Wheel Motor Support   FrontBack (Autodesk Fusion 360 design; units mm, degrees)
Autodesk Fusion 360 part; units mm, degrees
note: some values were not read from the file. Chosen so that the rebuilt part matches the saved one: which pieces of a blend or face edit are solid. Set by a fixed rule: which sketch regions a step uses.
sketch "Sketch1" plane through (0, 0, 0) normal (0, 0, 1) x (1, 0, 0)
  circle A0 centre (0, 0) radius 15.5 construction
  circle A1 centre (0, 0) radius 18.9
  circle A2 centre (0, 0) radius 20.9
  line L0 (-18.9, 0) -> (18.9, 0) construction
  circle A3 centre (-15.5, 0) radius 1.6
  circle A4 centre (15.5, 0) radius 1.6
  circle A5 centre (7.75, -13.4234) radius 1.6
  circle A6 centre (-7.75, -13.4234) radius 1.6
  circle A7 centre (7.75, 13.4234) radius 1.6
  circle A8 centre (-7.75, 13.4234) radius 1.6
  line L1 (0, 18.9) -> (0, -19.1322) construction
  circle A9 centre (0, -7) radius 6.25
  circle A10 centre (0, 7) radius 6.25
  line L2 (6.25, 7) -> (6.25, -7)
  line L3 (-6.25, 7) -> (-6.25, -7)
  dimension "d1" = 31
  dimension "d2" = 37.8
  dimension "d3" = 2
  dimension "d4" = 3.2
  dimension "d5" = 3.2
  dimension "d6" = 3.2
  dimension "d7" = 3.2
  dimension "d8" = 3.2
  dimension "d9" = 3.2
  dimension "d10" = 15.5
  dimension "d11" = 15.5
  dimension "d12" = 15.5
  dimension "d13" = 15.5
  dimension "d14" = 15.5
  dimension "d15" = 12.5
  dimension "d16" = 7
  dimension "d32" = 12.5
  dimension "d33" = 7
  constraint coincident A0.centre A1.centre
  constraint concentric A0 A1
  constraint horizontal L0
  constraint coincident A1 L0.end
  constraint coincident A1 L0.start
  constraint coincident A0.centre L0
  constraint coincident A0 A3.centre
  constraint coincident L0 A3.centre
  constraint coincident A0 A4.centre
  constraint coincident L0 A4.centre
  constraint coincident A0 A5.centre
  constraint coincident A0 A6.centre
  constraint coincident A0 A7.centre
  constraint coincident A0 A8.centre
  constraint coincident A1 L1.start
  constraint perpendicular L0 L1
  constraint coincident A0.centre L1
  constraint coincident A10 L2.start
  constraint coincident A9 L2.end
  constraint tangent A9 L2
  constraint vertical L2
  constraint coincident L1 A10.centre
  constraint coincident L1 A9.centre
  constraint coincident A10 L3.start
  constraint coincident A9 L3.end
  constraint tangent A9 L3
  constraint tangent A10 L3
  measures "d1" diameter of A0
  measures "d2" diameter of A1
  measures "d3" distance of A1 A2
  measures "d4" diameter of A3
  measures "d5" diameter of A4
  measures "d6" diameter of A5
  measures "d7" diameter of A6
  measures "d8" diameter of A7
  measures "d9" diameter of A8
  measures "d10" distance of A3.centre A6.centre
  measures "d11" distance of A4.centre A5.centre
  measures "d12" distance of A5.centre A6.centre
  measures "d13" distance of A4.centre A7.centre
  measures "d14" distance of A3.centre A8.centre
  measures "d15" diameter of A9
  measures "d16" distance of A0.centre A9.centre
  measures "d32" diameter of A10
  measures "d33" distance of A0.centre A10.centre
extrude "Extrude1" add sketch "Sketch1" along normal blind 3 contours A1 makes body 1
extrude "Extrude2" add sketch "Sketch1" along normal blind 75 contours A2 bodies 1
ref_plane "WorkPlane2" through (0, 20.9, 47.783) normal (0, 1, 0) x (1, 0, 0)
sketch "Sketch7" plane through (0, 20.9, 47.3257) normal (0, 1, 0) x (1, 0, 0)
  line L0 (-20.9, -27.6743) -> (20.9, -27.6743)
  line L1 (-10, -27.6743) -> (10, -27.6743)
  line L2 (10, -27.6743) -> (10, 17.3257)
  line L3 (10, 17.3257) -> (-10, 17.3257)
  line L4 (-10, 17.3257) -> (-10, -27.6743)
  line L5 (-10, -27.6743) -> (10, 17.3257) construction
  line L6 (10, -27.6743) -> (-10, 17.3257) construction
  line L7 (0, -27.6743) -> (0, -5.1743) construction
  point P0 (0, -5.1743)
  dimension "d137" = 45
  dimension "d138" = 20
  constraint perpendicular L1 L2
  constraint parallel L1 L3
  constraint parallel L2 L4
  constraint horizontal L1
  constraint coincident L0 L1.start
  constraint coincident L5 P0
  constraint coincident L6 P0
  constraint midpoint L0 L7.start
  constraint coincident P0 L7.end
  constraint vertical L7
  measures "d137" distance of L1.end L2.end
  measures "d138" distance of L1.start L1.end
extrude "Extrude8" add sketch "Sketch7" against normal blind 5 bodies 1
extrude "Extrude9" cut 1 faces at (8.8, 0, 3) along direction (0, 0, 1) through all on bodies 1 bodies 1
fillet "Fillet9" radius 130 2 edges at (-10, 18.3524, 52.5) (10, 18.3524, 52.5) on bodies 1
sketch "Sketch9" plane through (0, 0, 75) normal (0, 0, 1) x (-1, 0, 0)
  arc A0 (15.814, -13.6648) -> (10, -20.9) centre (114.1784, -98.6615) ccw
  arc A1 (15.814, -13.6648) -> (-15.814, -13.6648) centre (0, 0) ccw
  arc A2 (-10, -20.9) -> (-15.814, -13.6648) centre (-114.1784, -98.6615) ccw
  circle A3 centre (0, 0) radius 18.9
  line L0 (0, 0) -> (0, 20.9) construction
  line L1 (0, 0) -> (-14.7785, 14.7785)
  line L2 (0, 0) -> (14.7785, 14.7785)
  line L3 (-10, -20.9) -> (10, -20.9)
  dimension "d155" = 45
  dimension "d156" = 45
  constraint coincident A1.centre A3.centre
  constraint vertical L0
  constraint midpoint A1 L0.end
  constraint coincident A1 L1.end
  constraint coincident A1 L2.end
  measures "d155" angle of L0 L1
  measures "d156" angle of L0 L2
extrude "Extrude10" cut sketch "Sketch9" against normal blind 20 contours A1 A3 L1 L2 bodies 1
sketch "Sketch12" plane through (0, 0, 0) normal (1, 0, 0) x (0, 1, 0)
  line L0 (20.9, 30) -> (20.9, 75)
  line L1 (20.9, 75) -> (20.9, 51.5)
  line L2 (20.9, 51.5) -> (32.4272, 58.3142)
  line L3 (43, 61.5) -> (55.5, 61.5)
  line L4 (55.5, 61.5) -> (55.5, 82)
  line L5 (55.5, 82) -> (43, 82)
  line L6 (43, 61.5) -> (32.4272, 58.3142)
  line L7 (27.4533, 80.8489) -> (43, 82)
  line L8 (13.6648, 75) -> (20.9, 75)
  line L9 (27.4533, 80.8489) -> (19.4, 75)
  line L10 (19.4, 75) -> (20.9, 75)
  line L11 (100.5, 34) -> (79.5, 34)
  line L12 (79.5, 34) -> (73.4531, 50.9539)
  line L13 (73.4531, 50.9539) -> (65.3042, 58.3427)
  line L14 (65.3042, 58.3427) -> (55.5, 61.5)
  line L15 (100.5, 34) -> (96.8275, 51.6214)
  line L16 (96.8275, 51.6214) -> (88.5934, 64.8196)
  line L17 (88.5934, 64.8196) -> (76.9028, 75.9256)
  line L18 (76.9028, 75.9256) -> (67.1119, 80.748)
  line L19 (67.1119, 80.748) -> (55.5, 82)
  dimension "d163" = 23.5
  dimension "d164" = 12.5
  dimension "d165" = 20.5
  dimension "d166" = 12.5
  dimension "d168" = 34.6
  dimension "d169" = 1.5
  dimension "d172" = 13.5
  dimension "d179" = 45
  dimension "d180" = 21
  dimension "d181" = 18
  dimension "d182" = 11
  dimension "d183" = 10.3
  dimension "d184" = 27.5
  dimension "d185" = 18
  constraint coincident L0.end L1.start
  constraint parallel L0 L1
  constraint horizontal L3
  constraint perpendicular L3 L4
  constraint perpendicular L4 L5
  constraint coincident L8 L9.end
  constraint perpendicular L0 L10
  constraint horizontal L11
  measures "d163" distance of L0.end L1.end
  measures "d164" distance of L3.start L3.end
  measures "d165" distance of L3.end L4.end
  measures "d166" distance of L4.end L5.end
  measures "d168" distance of L0.end L4
  measures "d169" distance of L9.end L0.end
  measures "d172" vertical distance of L3.end L0.end
  measures "d179" horizontal distance of L3.end L11.start
  measures "d180" distance of L11.start L11.end
  measures "d181" distance of L11.end L12.end
  measures "d182" distance of L12.end L13.end
  measures "d183" distance of L3.end L13.end
  measures "d184" vertical distance of L3.end L11.end
  measures "d185" distance of L11.start L15.end
extrude "Extrude12" add sketch "Sketch12" along normal mid plane 20 contours L0 L1 L2 L3 L4 L5 L6 L7 L8 L9 L10 bodies 1
extrude "Extrude14" add sketch "Sketch12" along normal mid plane 20 separate body contours L4 L11 L12 L13 L14 L15 L16 L17 L18 L19 makes body 2
sketch "Sketch13" plane through (0, 55.5, 0) normal (0, 1, 0) x (-1, 0, 0)
  line L0 (10, 82) -> (-10, 82)
  line L1 (-10, 82) -> (-10, 61.5)
  line L2 (-10, 61.5) -> (10, 61.5)
  line L3 (10, 61.5) -> (10, 82)
  line L4 (10, 82) -> (-10, 61.5) construction
  line L5 (5.1, 77.85) -> (-5.1, 77.85)
  line L6 (-5.1, 77.85) -> (-5.1, 65.65)
  line L7 (-5.1, 65.65) -> (5.1, 65.65)
  line L8 (5.1, 65.65) -> (5.1, 77.85)
  line L9 (5.1, 77.85) -> (-5.1, 65.65) construction
  line L10 (-5.1, 77.85) -> (5.1, 65.65) construction
  point P0 (0, 71.75)
  dimension "d173" = 12.2
  dimension "d174" = 10.2
  constraint coincident L0.start L3.end
  constraint coincident L1.end L2.start
  constraint perpendicular L5 L6
  constraint parallel L5 L7
  constraint parallel L6 L8
  constraint horizontal L5
  constraint coincident L9 P0
  constraint coincident L10 P0
  constraint midpoint L4 P0
  measures "d173" distance of L5.end L6.end
  measures "d174" distance of L6.end L7.end
extrude "Extrude13" cut sketch "Sketch13" against normal blind 21 contours L5 L6 L7 L8 bodies 1
sketch "Sketch14" plane through (0, 55.5, 0) normal (0, -1, 0) x (1, 0, 0)
  line L0 (-10, 61.5) -> (10, 61.5)
  line L1 (10, 61.5) -> (10, 82)
  line L2 (10, 82) -> (-10, 82)
  line L3 (-10, 82) -> (-10, 61.5)
  line L4 (10, 82) -> (-10, 61.5) construction
  line L5 (5, 65.75) -> (-5, 65.75)
  line L6 (-5, 65.75) -> (-5, 77.75)
  line L7 (-5, 77.75) -> (5, 77.75)
  line L8 (5, 77.75) -> (5, 65.75)
  line L9 (5, 65.75) -> (-5, 77.75) construction
  line L10 (-5, 65.75) -> (5, 77.75) construction
  point P0 (0, 71.75)
  dimension "d188" = 10
  dimension "d189" = 12
  constraint coincident L1.end L2.start
  constraint coincident L0.start L3.end
  constraint perpendicular L5 L6
  constraint parallel L5 L7
  constraint parallel L6 L8
  constraint horizontal L5
  constraint coincident L9 P0
  constraint coincident L10 P0
  constraint midpoint L4 P0
  measures "d188" distance of L6.end L7.end
  measures "d189" distance of L5.end L6.end
extrude "Extrude15" add sketch "Sketch14" along normal blind 20 contours L5 L6 L7 L8 bodies 2
fillet "Fillet10" radius 17.5 1 edges at (0, 20.9, 51.5) on bodies 1
fillet "Fillet11" radius 1.5 14 edges at (10, 49.25, 61.5) (10, 37.7136, 59.9071) (10, 49.25, 82) (10, 35.2267, 81.4244) (10, 23.4267, 77.9244) (10, 30.9609, 57.4474) (10, 23.1998, 50.1879) (-10, 49.25, 61.5) (-10, 37.7136, 59.9071) (-10, 30.9609, 57.4474) (-10, 23.1998, 50.1879) (-10, 23.4267, 77.9244) (-10, 35.2267, 81.4244) (-10, 49.25, 82) on bodies 1 2
fillet "Fillet11" radius 1.5 16 edges at (-10, 61.306, 81.374) (-10, 72.0074, 78.3368) (-10, 82.7481, 70.3726) (-10, 92.7104, 58.2205) (-10, 98.6637, 42.8107) (-10, 76.4766, 42.477) (-10, 69.3786, 54.6483) (-10, 60.4021, 59.9214) (10, 60.4021, 59.9214) (10, 69.3786, 54.6483) (10, 76.4766, 42.477) (10, 61.306, 81.374) (10, 72.0074, 78.3368) (10, 82.7481, 70.3726) (10, 92.7104, 58.2205) (10, 98.6637, 42.8107) on bodies 1 2
ref_plane "WorkPlane4" through (0, 100.5, 34) normal (0, 1, 0) x (-1, 0, 0)
sketch "Sketch15" plane through (0, 100.5, 34) normal (0, 1, 0) x (1, 0, 0)
  line L0 (0, 0) -> (0, 43.3) construction
  circle A0 centre (0, 43.3) radius 29
  line L1 (10, 0) -> (25.669, 29.8056)
  line L2 (-10, 0) -> (-25.669, 29.8056)
  circle A1 centre (0, 43.3) radius 23.5
  line L3 (-10, 0) -> (10, 0)
  circle A2 centre (0, 43.3) radius 6
  point P0 (-10, 0)
  point P1 (10, 0)
  point P2 (0, 43.3)
  dimension "d194" = 43.3
  dimension "d195" = 58
  dimension "d196" = 47
  dimension "d207" = 12
  constraint coincident L0.start origin
  constraint vertical L0
  constraint coincident L0.end A0.centre
  constraint coincident P1 L1.start
  constraint coincident A0 L1.end
  constraint tangent A0 L1
  constraint coincident P0 L2.start
  constraint coincident A0 L2.end
  constraint tangent A0 L2
  constraint concentric A0 A1
  constraint coincident P2 L0.end
  measures "d194" distance of L0.start L0.end
  measures "d195" diameter of A0
  measures "d196" diameter of A1
  measures "d207" diameter of A2
extrude "Extrude18" add sketch "Sketch15" against normal blind 21 contours A0 | A0 L1 L2 L3 | A1 bodies 2
sketch "Sketch16" plane through (0, 0, 0) normal (1, 0, 0) x (0, 1, 0)
  line L0 (100.5, -38.3) -> (100.5, 19.7)
  line L1 (79.5, 4.1944) -> (79.5, -38.3)
  line L2 (79.5, 4.1944) -> (79.5, 34)
  line L3 (100.5, 34) -> (100.5, 4.1944)
  line L4 (79.5, -38.3) -> (100.5, -38.3) construction
  line L5 (90, -38.3) -> (79.5, 19.0972)
  line L6 (79.5, -38.3) -> (90, -38.3)
  constraint coincident L1.end L4.start
  constraint coincident L0.start L4.end
  constraint midpoint L4 L5.start
  constraint midpoint L2 L5.end
extrude "Extrude19" cut sketch "Sketch16" along normal through all and the other way through all bodies 2
extrude "Extrude20" add sketch "Sketch15" against normal blind 21 contours A1 bodies 2
sketch "Sketch17" plane through (0, 79.5, 0) normal (0, -1, 0) x (1, 0, 0)
  circle A0 centre (0, -9.3) radius 6
  circle A1 centre (0, -9.3) radius 23.5
  line L0 (-5.7735, 0.7) -> (-11.547, -9.3)
  line L1 (-11.547, -9.3) -> (-5.7735, -19.3)
  line L2 (-5.7735, -19.3) -> (5.7735, -19.3)
  line L3 (5.7735, -19.3) -> (11.547, -9.3)
  line L4 (11.547, -9.3) -> (5.7735, 0.7)
  line L5 (5.7735, 0.7) -> (-5.7735, 0.7)
  point P0 (0, -9.3)
  dimension "d208" = 10
  constraint coincident P0 A0.centre
  measures "d208" distance of P0 L5
extrude "Extrude21" cut sketch "Sketch17" against normal blind 5 contours L0 L1 L2 L3 L4 L5 bodies 2
named bodies: "WMS - FrontBack - bas", "WMS - FrontBack - haut"
